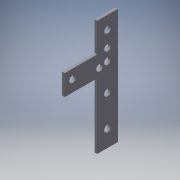
# Autodesk Inventor part: Mounting_wall_3
Saved by Autodesk Inventor 2017 (Build 210142000, 142)
## iProperties
Created: 2017-11-15
Part Number: Mounting_wall_3
Material: Generic
Document SubType Name: Modeling
Designer: julie
Density: 1 g/cm^3
Appearance: Default
Author: julie
Autodesk Inventor part; units mm, degrees
ref_plane "YZ Plane" through (0, 0, 0) normal (1, 0, 0) x (0, 1, 0)
ref_plane "XZ Plane" through (0, 0, 0) normal (0, 1, 0) x (-1, 0, 0)
ref_plane "XY Plane" through (0, 0, 0) normal (0, 0, 1) x (1, 0, 0)
sketch "Sketch1" plane through (0, 0, 0) normal (1, 0, 0) x (0, 1, 0)
  line L0 (0, 0) -> (16, 0)
  line L1 (16, 0) -> (16, -100)
  line L2 (16, -100) -> (0, -100)
  line L3 (0, -10) -> (0, -10)
  line L4 (0, -10) -> (0, -25)
  line L5 (0, -25) -> (0, -25)
  line L6 (0, -90) -> (0, -90)
  line L7 (0, -90) -> (0, -75)
  line L8 (0, -75) -> (0, -75)
  line L9 (0, -10) -> (0, 0)
  line L10 (0, -100) -> (0, -90)
  line L11 (0, -75) -> (0, -25)
  dimension "d0" = 16
  dimension "d1" = 100
  dimension "d2" = 0
  dimension "d3" = 15
  dimension "d4" = 10
  dimension "d5" = 15
  dimension "d6" = 10
  dimension "d10" = 0
  dimension "d11" = 0
  dimension "d12" = 0
  constraints: 24 end point, 9 perpendicular, 4 parallel, 3 horizontal
  measures "d0" distance of L1.end L2.end
  measures "d1" distance of L0.end L1.end
  measures "d2" distance of L3.start L3.end
  measures "d3" distance of L3.end L4.end
  measures "d4" distance from line of L0.start L3
  measures "d5" distance of L6.end L7.end
  measures "d6" distance between parallel lines of L2 L6
  measures "d10" distance of L6.start L6.end
  measures "d11" distance from line of L0.start L11
  measures "d12" distance of L7.end L8.end
extrude "Extrusion1" add sketch "Sketch1" along normal blind 2
sketch "Sketch5" plane through (2, 0, 0) normal (1, 0, 0) x (0, 0, -1)
  line L0 (0, 0) -> (100, 0) projected
  circle A0 centre (63.5, -19) radius 2.5 projected
  line L1 (56.5, 0) -> (72.5, 0)
  line L2 (72.5, 0) -> (72.5, -25)
  line L3 (72.5, -25) -> (56.5, -25)
  line L4 (56.5, -25) -> (56.5, 0)
  circle A1 centre (66.2831, 1.8148) radius 2.5
  circle A2 centre (56, 8) radius 6 construction
  circle A3 centre (63.5, -19) radius 15 construction
  circle A4 centre (66.2831, 1.8148) radius 6 construction
  dimension "d44" = 16
  dimension "d45" = 25
  dimension "d46" = 9
  dimension "d52" = 5
  dimension "d56" = 12
  dimension "d57" = 30
  dimension "d58" = 12
  constraints: 8 end point, 4 centre point, 3 coincident, 2 parallel, 2 tangent, 1 horizontal, 1 perpendicular, 1 point on line
  measures "d44" distance of L2.end L3.end
  measures "d45" distance of L1.end L2.end
  measures "d46" distance from line of L2 A0.centre
  measures "d52" diameter of A1
  measures "d56" diameter of A2
  measures "d57" diameter of A3
  measures "d58" diameter of A4
extrude "Extrusion6" add sketch "Sketch5" against normal blind 2 contours L0 A1 L2 L3 L4 | L0 A1 picked at (65.8534, -0.1091)
sketch "Sketch7" plane through (2, 0, 0) normal (1, 0, 0) x (0, 0, -1)
  circle A0 centre (44, 8) radius 2.5 projected
  circle A1 centre (56, 8) radius 2.5 projected
  circle A2 centre (66.2831, 1.8148) radius 2.5 projected
  circle A3 centre (63.5, -19) radius 2.5 projected
  circle A4 centre (44, 8) radius 2.5
  circle A5 centre (56, 8) radius 2.5
  circle A6 centre (66.2831, 1.8148) radius 2.5
  circle A7 centre (63.5, -19) radius 2.5 projected
  circle A8 centre (63.5, -19) radius 2.5
  point P0 (0, 0)
  dimension "d59" = 5
  dimension "d60" = 5
  dimension "d61" = 5
  dimension "d62" = 5
  constraints: 4 centre point, 4 coincident
  measures "d59" diameter of A4
  measures "d60" diameter of A5
  measures "d61" diameter of A6
  measures "d62" diameter of A8
extrude "Extrusion8" cut sketch "Sketch7" against normal blind 10 contours A0 | A1 | A2
sketch "Sketch8" plane through (2, 0, 0) normal (1, 0, 0) x (0, 0, -1)
  circle A0 centre (44, 8) radius 2.5 projected
  line L0 (0, 0) -> (56.5, 0) projected
  line L1 (0, 16) -> (0, 0) projected
  line L2 (100, 16) -> (0, 16) projected
  line L3 (56.5, 0) -> (0, 0) projected
  line L4 (34, 0) -> (0, 0)
  line L5 (0, 0) -> (0, 16)
  line L6 (0, 16) -> (34, 16)
  line L7 (34, 16) -> (34, 0)
  dimension "d65" = 10
  constraints: 8 end point, 2 parallel, 1 horizontal, 1 perpendicular, 1 point on line
  measures "d65" distance from line of L7 A0.centre
extrude "Extrusion9" cut sketch "Sketch8" against normal blind 10 contours L1 L2 L7 L0
sketch "Sketch9" plane through (2, 0, 0) normal (1, 0, 0) x (0, 0, -1)
  circle A0 centre (56, 8) radius 2.5 projected
  circle A1 centre (66.2831, 1.8148) radius 2.5 projected
  circle A2 centre (65, 7.8652) radius 2.5
  circle A3 centre (86, 7.8652) radius 2.5
  circle A4 centre (44, 8) radius 2.5 projected
  point P0 (0, 0)
  dimension "d68" = 5
  dimension "d71" = 5
  dimension "d72" = 21
  dimension "d76" = 21
  dimension "d77" = 6.0505
  dimension "d78" = 6.0505
  constraints: 2 centre point
  measures "d68" diameter of A2
  measures "d71" diameter of A3
  measures "d72" distance of A2.centre A3.centre
  measures "d76" horizontal distance of A4.centre A2.centre
  measures "d77" vertical distance of A1.centre A2.centre
  measures "d78" vertical distance of A1.centre A3.centre
extrude "Extrusion10" cut sketch "Sketch9" against normal blind 10 contours A2 | A3
sketch "Sketch10" plane through (0, 0, 0) normal (-1, 0, 0) x (0, 0, 1)
  line L0 (-124, 20) -> (-103.2154, 17) projected
  line L1 (-124, -1) -> (-124, 20) projected
  line L2 (-102, -1) -> (-124, -1) projected
  line L3 (-102, -1) -> (-102, 17) projected
  line L4 (-103.2154, 17) -> (-102, 17) projected
  circle A0 centre (-65, 7.8652) radius 2.5 projected
  circle A1 centre (-86, 7.8652) radius 2.5 projected
  line L5 (-34, 0) -> (-34, 16) projected
  line L6 (-34, 16) -> (-100, 16) projected
  line L7 (-100, 16) -> (-100, 0) projected
  line L8 (-100, 0) -> (-72.5, 0) projected
  line L9 (-72.5, 0) -> (-72.5, -25) projected
  line L10 (-72.5, -25) -> (-56.5, -25) projected
  line L11 (-56.5, -25) -> (-56.5, 0) projected
  line L12 (-56.5, 0) -> (-34, 0) projected
  circle A2 centre (-63.5, -19) radius 2.5 projected
  circle A3 centre (-66.2831, 1.8148) radius 2.5 projected
  circle A4 centre (-44, 8) radius 2.5 projected
  circle A5 centre (-56, 8) radius 2.5 projected
  line L13 (-100, 16) -> (-123, 16)
  line L14 (-123, 16) -> (-123, 0)
  line L15 (-123, 0) -> (-100, 0)
  line L16 (-100, 0) -> (-100, 16)
  point P0 (0, 0)
  dimension "d79" = 23
  constraints: 8 end point, 2 parallel, 1 horizontal, 1 perpendicular
  measures "d79" distance of L15.end L14.end
extrude "Extrusion11" add sketch "Sketch10" against normal blind 2 contours L13 L7 L15 L3 | L3 L15 L14 L13
sketch "Sketch11" plane through (2, 0, 0) normal (1, 0, 0) x (0, 0, -1)
  circle A0 centre (110, 7.8652) radius 2.5 projected
  circle A1 centre (110, 7.8652) radius 2.5
  point P0 (0, 0)
  dimension "d82" = 5
  constraints: 1 centre point, 1 coincident
  measures "d82" diameter of A1
extrude "Extrusion12" cut sketch "Sketch11" against normal blind 10
equation "\"d78\" = d77"
body "Solid1"
